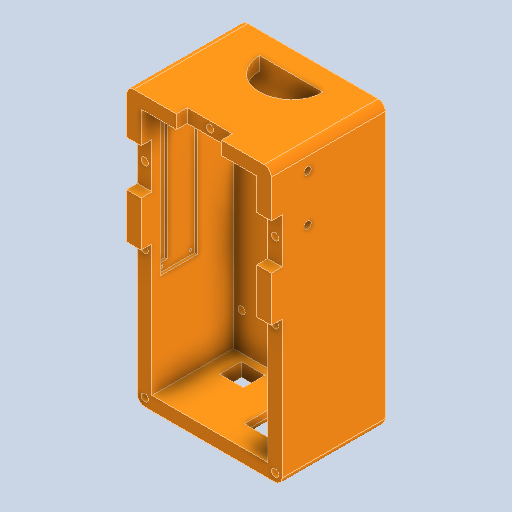
# Autodesk Inventor part: Caja para Electrónica
Saved by Autodesk Inventor 2026 (Build 300175050, 175E)
## iProperties
Created: 2026-02-09
Part Number: Caja para Electrónica
Material: Genérico
Document SubType Name: Modeling
Designer: bello
Density: 1 g/cm^3
Appearance: Naranja
Author: bello
Autodesk Inventor part; units mm, degrees
ref_plane "YZ Plane" through (0, 0, 0) normal (1, 0, 0) x (0, 1, 0)
ref_plane "XZ Plane" through (0, 0, 0) normal (0, 1, 0) x (-1, 0, 0)
ref_plane "XY Plane" through (0, 0, 0) normal (0, 0, 1) x (1, 0, 0)
sketch "Boceto1" plane through (0, 0, 0) normal (0, 0, 1) x (1, 0, 0)
  line L0 (0, 0) -> (80, 0)
  line L1 (80, 0) -> (80, -155)
  line L2 (80, -155) -> (0, -155)
  line L3 (0, -155) -> (0, 0)
  dimension "d0" = 155
  dimension "d1" = 80
  constraints: 8 end point, 2 parallel, 1 horizontal, 1 perpendicular
  measures "d0" distance of L0.end L1.end
  measures "d1" distance of L0.start L0.end
extrude "Extrusión1" add sketch "Boceto1" along normal blind 82
sketch "Boceto2" plane through (0, 0, 82) normal (0, 0, 1) x (1, 0, 0)
  line L0 (8, -7.5) -> (72, -7.5)
  line L1 (72, -7.5) -> (72, -147.5)
  line L2 (72, -147.5) -> (8, -147.5)
  line L3 (8, -147.5) -> (8, -7.5)
  line L4 (80, -155) -> (80, 0) projected
  line L5 (0, 0) -> (0, -155) projected
  line L6 (80, 0) -> (0, 0) projected
  line L7 (0, -155) -> (80, -155) projected
  dimension "d4" = 8
  dimension "d5" = 8
  dimension "d6" = 7.5
  dimension "d7" = 7.5
  dimension "d8" = 64
  dimension "d9" = 140
  constraints: 8 end point, 2 parallel, 1 horizontal, 1 perpendicular
  measures "d4" distance between parallel lines of L4 L1
  measures "d5" distance between parallel lines of L5 L3
  measures "d6" distance between parallel lines of L6 L0
  measures "d7" distance between parallel lines of L7 L2
  measures "d8" distance between parallel lines of L1 L3
  measures "d9" distance between parallel lines of L2 L0
extrude "Extrusión2" cut sketch "Boceto2" against normal blind 70 contours L0 L1 L2 L3
sketch "Boceto3" plane through (0, 0, 12) normal (0, 0, 1) x (1, 0, 0)
  line L0 (72, -147.5) -> (8, -147.5) projected
  line L1 (8, -147.5) -> (8, -7.5) projected
  line L2 (72, -7.5) -> (72, -147.5) projected
  line L3 (10, -142) -> (70, -142)
  circle A0 centre (12.5, -127) radius 2
  circle A1 centre (60.5, -128) radius 2
  circle A2 centre (60.5, -46.5) radius 2
  point P0 (0, 0)
  dimension "d20" = 60
  dimension "d21" = 2
  dimension "d22" = 2
  dimension "d23" = 5.5
  dimension "d24" = 15
  dimension "d25" = 14
  dimension "d26" = 4.5
  dimension "d27" = 11.5
  dimension "d28" = 95.5
  dimension "d29" = 11.5
  dimension "d30" = 4
  constraints: 3 centre point, 2 end point, 2 equal radius, 1 horizontal
  measures "d20" distance of L3.start L3.end
  measures "d21" distance from line of L1 L3.start
  measures "d22" distance from line of L2 L3.end
  measures "d23" distance between parallel lines of L0 L3
  measures "d24" distance from line of L3 A0.centre
  measures "d25" distance from line of L3 A1.centre
  measures "d26" distance from line of L1 A0.centre
  measures "d27" distance from line of L2 A1.centre
  measures "d28" distance from line of L3 A2.centre
  measures "d29" distance from line of L2 A2.centre
  measures "d30" diameter of A2
extrude "Extrusión3" cut sketch "Boceto3" against normal blind 6.7
sketch "Boceto4" plane through (0, 0, 12) normal (0, 0, 1) x (1, 0, 0)
  line L0 (40, 12.201) -> (40, -183.6096)
  circle A0 centre (40, -57.5) radius 3
  circle A1 centre (40, -117.5) radius 3
  line L1 (72, -147.5) -> (8, -147.5) projected
  line L2 (0, -155) -> (80, -155) projected
  point P0 (0, 0)
  point P1 (40, -155)
  point P2 (40, -155)
  dimension "d33" = 60
  dimension "d34" = 6
  dimension "d35" = 30
  dimension "d103" = 0
  constraints: 2 centre point, 2 end point, 2 midpoint, 2 point on line, 1 equal radius
  measures "d33" distance of A1.centre A0.centre
  measures "d34" diameter of A0
  measures "d35" distance from line of L1 A1.centre
  measures "d103" distance from line of point (40, -155) L0
extrude "Extrusión4" cut sketch "Boceto4" against normal through all
sketch "Boceto5" plane through (0, 0, 12) normal (0, 0, 1) x (1, 0, 0)
  circle A0 centre (40, -57.5) radius 3 projected
  line L0 (45.9467, -57.5) -> (42.9734, -62.65)
  line L1 (42.9734, -62.65) -> (37.0266, -62.65)
  line L2 (37.0266, -62.65) -> (34.0533, -57.5)
  line L3 (34.0533, -57.5) -> (37.0266, -52.35)
  line L4 (37.0266, -52.35) -> (42.9734, -52.35)
  line L5 (42.9734, -52.35) -> (45.9467, -57.5)
  circle A1 centre (40, -117.5) radius 3 projected
  line L6 (45.9467, -117.5) -> (42.9734, -122.65)
  line L7 (42.9734, -122.65) -> (37.0266, -122.65)
  line L8 (37.0266, -122.65) -> (34.0533, -117.5)
  line L9 (34.0533, -117.5) -> (37.0266, -112.35)
  line L10 (37.0266, -112.35) -> (42.9734, -112.35)
  line L11 (42.9734, -112.35) -> (45.9467, -117.5)
  point P0 (0, 0)
  dimension "d38" = 10.3
  constraints: 24 end point, 2 coincident, 1 parallel, 26 other
  measures "d38" distance between parallel lines of L1 L4
extrude "Extrusión5" cut sketch "Boceto5" against normal blind 6 contours A0 | L0 L1 L2 L3 L4 L5 | A1 | L6 L7 L8 L9 L10 L11
sketch "Boceto6" plane through (0, -155, 0) normal (0, -1, 0) x (1, 0, 0)
  line L0 (0, 0) -> (80, 0) projected
  line L1 (72, 12) -> (8, 12) projected
  line L2 (16.5, 16) -> (29.5, 16)
  line L3 (16.5, 28) -> (29.5, 28)
  line L4 (10, 12) -> (10, 44.9628)
  line L5 (70, 12) -> (70, 46.4487)
  line L6 (8, 82) -> (8, 12) projected
  line L7 (72, 82) -> (72, 12) projected
  line L8 (16.5, 28) -> (16.5, 16)
  line L9 (29.5, 28) -> (29.5, 16)
  line L10 (47, 45) -> (68.5, 45)
  line L11 (47, 28.5) -> (68.5, 28.5)
  line L12 (47, 28.5) -> (47, 45)
  line L13 (68.5, 28.5) -> (68.5, 45)
  point P0 (23, 16)
  dimension "d41" = 12
  dimension "d42" = 4
  dimension "d43" = 16
  dimension "d44" = 2
  dimension "d45" = 2
  dimension "d46" = 13
  dimension "d47" = 13
  dimension "d48" = 6.5
  dimension "d49" = 6.5
  dimension "d50" = 12
  dimension "d53" = 33
  dimension "d54" = 16.5
  dimension "d55" = 21.5
  dimension "d56" = 1.5
  dimension "d57" = 1.5
  dimension "d58" = 16.5
  constraints: 20 end point, 4 horizontal, 2 point on line, 2 vertical, 1 midpoint, 1 parallel
  measures "d41" distance between parallel lines of L0 L1
  measures "d42" distance between parallel lines of L1 L2
  measures "d43" distance between parallel lines of L1 L3
  measures "d44" distance between parallel lines of L6 L4
  measures "d45" distance between parallel lines of L7 L5
  measures "d46" distance of L3.start L3.end
  measures "d47" distance of L2.start L2.end
  measures "d48" distance from line of L4 L3.start
  measures "d49" distance from line of L4 L2.start
  measures "d50" distance from line of point (23, 16) L3
  measures "d53" distance between parallel lines of L1 L10
  measures "d54" distance between parallel lines of L1 L11
  measures "d55" distance of L10.start L10.end
  measures "d56" distance from line of L5 L10.end
  measures "d57" distance from line of L5 L11.end
  measures "d58" distance between parallel lines of L10 L11
extrude "Extrusión6" cut sketch "Boceto6" against normal up to surface (7.5 mm away)
fillet "Empalme1" radius 4 4 edges at (47, -155, 36.75) (57.75, -155, 45) (68.5, -155, 36.75) (57.75, -155, 28.5)
sketch "Boceto8" plane through (72, -147.5, 82) normal (-1, 0, 0) x (0, 0, 1)
  line L0 (-50, 126.4237) -> (-50, 59.6822)
  line L1 (-70, 0) -> (-70, 140) projected
  circle A0 centre (-39, 136.5) radius 2
  circle A1 centre (-39, 110.5) radius 2
  line L2 (-54.9354, 5.5) -> (-15.6963, 5.5)
  line L3 (0, 0) -> (-70, 0) projected
  line L4 (-50, 108) -> (-15.6963, 108)
  line L5 (-50, 139) -> (-21.6523, 139)
  point P0 (-82, 147.5)
  dimension "d60" = 20
  dimension "d61" = 4
  dimension "d62" = 11
  dimension "d63" = 11
  dimension "d64" = 5.5
  dimension "d65" = 102.5
  dimension "d66" = 2.5
  dimension "d67" = 31
  dimension "d68" = 2.5
  constraints: 8 end point, 3 horizontal, 2 centre point, 2 point on line, 1 equal radius, 1 vertical
  measures "d60" distance between parallel lines of L1 L0
  measures "d61" diameter of A0
  measures "d62" distance from line of A0.centre L0
  measures "d63" distance from line of L0 A1.centre
  measures "d64" distance between parallel lines of L3 L2
  measures "d65" distance between parallel lines of L2 L4
  measures "d66" distance from line of L4 A1.centre
  measures "d67" distance between parallel lines of L4 L5
  measures "d68" distance from line of L5 A0.centre
extrude "Extrusión7" cut sketch "Boceto8" against normal through all
sketch "Boceto9" plane through (8, -147.5, 82) normal (1, 0, 0) x (0, 0, -1)
  line L0 (50, 55) -> (50, 136)
  line L1 (70, 140) -> (70, 0) projected
  line L2 (29.5, 55) -> (29.5, 136)
  line L3 (50, 55) -> (29.5, 55)
  line L4 (29.5, 136) -> (50, 136)
  point P0 (82, 147.5)
  point P1 (0, 140)
  point P2 (39.75, 55)
  dimension "d71" = 20
  dimension "d72" = 20.5
  dimension "d73" = 81
  dimension "d75" = 4
  dimension "d101" = 30.25
  constraints: 8 end point, 2 vertical, 1 horizontal, 1 midpoint, 1 parallel
  measures "d71" distance between parallel lines of L1 L0
  measures "d72" distance between parallel lines of L0 L2
  measures "d73" distance of L2.start L2.end
  measures "d75" vertical distance of point (0, 140) L2.end
  measures "d101" distance from line of L1 point (39.75, 55)
extrude "Extrusión8" cut sketch "Boceto9" against normal blind 1.5
sketch "Boceto10" plane through (6.5, -147.5, 82) normal (1, 0, 0) x (0, 0, -1)
  line L0 (35, 59.5) -> (35, 131.5)
  line L1 (35, 131.5) -> (31, 131.5)
  line L2 (31, 131.5) -> (31, 59.5)
  line L3 (31, 59.5) -> (35, 59.5)
  line L4 (29.5, 55) -> (29.5, 136) projected
  line L5 (29.5, 136) -> (50, 136) projected
  point P0 (82, 147.5)
  point P1 (29.5, 95.5)
  dimension "d79" = 72
  dimension "d80" = 1.5
  dimension "d81" = 4
  dimension "d83" = 36
  constraints: 8 end point, 2 perpendicular, 1 midpoint, 1 parallel, 1 vertical
  measures "d79" distance of L1.end L2.end
  measures "d80" distance between parallel lines of L2 L4
  measures "d81" distance between parallel lines of L0 L2
  measures "d83" distance from line of point (29.5, 95.5) L1
extrude "Extrusión9" cut sketch "Boceto10" against normal blind 1.5
sketch "Boceto11" plane through (6.5, -147.5, 82) normal (1, 0, 0) x (0, 0, -1)
  circle A0 centre (31.75, 57.5) radius 0.8
  circle A1 centre (47.75, 57.5) radius 0.8
  circle A2 centre (31.75, 133.5) radius 0.8
  circle A3 centre (47.75, 133.5) radius 0.8
  line L0 (50, 136) -> (50, 55) projected
  line L1 (50, 55) -> (29.5, 55) projected
  line L2 (29.5, 55) -> (29.5, 136) projected
  line L3 (29.5, 136) -> (50, 136) projected
  point P0 (82, 147.5)
  dimension "d86" = 1.6
  dimension "d88" = 2.25
  dimension "d89" = 2.25
  dimension "d91" = 2.5
  dimension "d92" = 2.25
  dimension "d93" = 2.5
  dimension "d94" = 2.5
  dimension "d95" = 2.5
  dimension "d96" = 2.25
  constraints: 4 centre point, 3 equal radius
  measures "d86" diameter of A0
  measures "d88" distance from line of L0 A1.centre
  measures "d89" distance from line of L0 A3.centre
  measures "d91" distance from line of L1 A0.centre
  measures "d92" distance from line of L2 A0.centre
  measures "d93" distance from line of L1 A1.centre
  measures "d94" distance from line of L3 A3.centre
  measures "d95" distance from line of L3 A2.centre
  measures "d96" distance from line of L2 A2.centre
extrude "Extrusión10" cut sketch "Boceto11" against normal blind 3.5 contours A0 | A1 | A2 | A3
sketch "Boceto12" plane through (0, 0, 82) normal (0, 0, 1) x (1, 0, 0)
  line L0 (0, -75) -> (80, -75)
  line L1 (0, -155) -> (80, -155) projected
  line L2 (0, -75) -> (0, -155)
  line L3 (0, -155) -> (80, -155)
  line L4 (80, -155) -> (80, -75)
  point P0 (0, 0)
  point P1 (40, -155)
  dimension "d99" = 80
  dimension "d100" = 40
  dimension "d104" = 80
  dimension "d105" = 80
  constraints: 8 end point, 2 perpendicular, 1 horizontal, 1 midpoint, 1 vertical
  measures "d99" distance of L0.start L0.end
  measures "d100" horizontal distance of point (40, -155) L0.start
  measures "d104" distance of L3.end L0.end
  measures "d105" distance between parallel lines of L1 L0
extrude "Extrusión11" cut sketch "Boceto12" against normal blind 25
sketch "Boceto13" plane through (8, -7.5, 82) normal (0, -1, 0) x (1, 0, 0)
  line L0 (0, -70) -> (64, -70) projected
  circle A0 centre (32, -70) radius 17.5
  point P0 (-8, -82)
  point P1 (49.5, -70)
  point P2 (14.5, -70)
  dimension "d108" = 35
  constraints: 1 centre point, 1 midpoint
  measures "d108" diameter of A0
extrude "Extrusión12" cut sketch "Boceto13" against normal through all contours A0 L0 picked at (31.4056, -58.945)
sketch "Boceto14" plane through (0, 0, 57) normal (0, 0, 1) x (1, 0, 0)
  circle A0 centre (4, -150.5) radius 2
  circle A1 centre (4, -79.5) radius 2
  circle A2 centre (76, -79.5) radius 2
  circle A3 centre (76, -150.5) radius 2
  line L0 (80, -155) -> (0, -155) projected
  line L1 (0, -155) -> (0, -75) projected
  line L2 (0, -75) -> (8, -75) projected
  line L3 (80, -75) -> (80, -155) projected
  line L4 (72, -75) -> (80, -75) projected
  point P0 (0, 0)
  dimension "d111" = 4
  dimension "d112" = 4.5
  dimension "d113" = 4
  dimension "d114" = 4.5
  dimension "d115" = 4
  dimension "d116" = 4
  dimension "d117" = 4.5
  dimension "d118" = 4
  dimension "d119" = 4.5
  constraints: 4 centre point, 3 equal radius
  measures "d111" diameter of A0
  measures "d112" distance from line of L0 A0.centre
  measures "d113" distance from line of L1 A0.centre
  measures "d114" distance from line of L2 A1.centre
  measures "d115" distance from line of L1 A1.centre
  measures "d116" distance from line of L3 A2.centre
  measures "d117" distance from line of L4 A2.centre
  measures "d118" distance from line of L3 A3.centre
  measures "d119" distance from line of L0 A3.centre
extrude "Extrusión13" cut sketch "Boceto14" against normal blind 6.7
sketch "Boceto15" plane through (0, 0, 82) normal (0, 0, 1) x (1, 0, 0)
  line L0 (0, 0) -> (0, -75) projected
  line L1 (72, -75) -> (80, -75) projected
  line L2 (0, 0) -> (80, 0)
  line L3 (80, 0) -> (80, -75)
  line L4 (80, -75) -> (0, -75)
  line L5 (0, -75) -> (0, 0)
  constraints: 8 end point, 2 parallel, 1 horizontal, 1 perpendicular
extrude "Extrusión14" cut sketch "Boceto15" against normal blind 19
fillet "Empalme2" radius 4 4 edges at (0, -155, 28.5) (80, -155, 28.5) (80, 0, 31.5) (0, 0, 31.5)
sketch "Boceto16" plane through (0, 0, 63) normal (0, 0, 1) x (1, 0, 0)
  line L0 (22.5, 0) -> (57.5, 0) projected
  line L1 (27.5, -7.5) -> (52.5, -7.5)
  line L2 (52.5, -7.5) -> (52.5, 0)
  line L3 (52.5, 0) -> (27.5, 0)
  line L4 (27.5, 0) -> (27.5, -7.5)
  line L5 (8, -147.5) -> (8, -7.5) projected
  line L6 (0, -25) -> (8, -25)
  line L7 (8, -25) -> (8, -50)
  line L8 (8, -50) -> (0, -50)
  line L9 (0, -50) -> (0, -25)
  line L10 (8, -75) -> (0, -75) projected
  line L11 (40, 16.6758) -> (40, -44.6226)
  line L12 (80, -25) -> (72, -25)
  line L13 (72, -25) -> (72, -50)
  line L14 (72, -50) -> (80, -50)
  line L15 (80, -50) -> (80, -25)
  point P0 (40, 0)
  dimension "d129" = 25
  dimension "d130" = 7.5
  dimension "d131" = 12.5
  dimension "d132" = 8
  dimension "d133" = 25
  dimension "d134" = 25
  constraints: 26 end point, 4 parallel, 4 symmetric about line, 2 horizontal, 2 perpendicular, 2 point on line, 1 midpoint, 1 vertical
  measures "d129" distance of L1.start L1.end
  measures "d130" distance of L1.end L2.end
  measures "d131" distance from line of point (40, 0) L4
  measures "d132" distance of L6.start L6.end
  measures "d133" distance of L8.end L6.start
  measures "d134" distance between parallel lines of L10 L8
extrude "Extrusión15" cut sketch "Boceto16" against normal blind 6
sketch "Boceto17" plane through (0, 0, 57) normal (0, 0, 1) x (1, 0, 0)
  circle A0 centre (40, -3.75) radius 2
  circle A1 centre (4, -37.5) radius 2
  line L0 (5, -77.7679) -> (5, -16) projected
  circle A2 centre (76, -37.5) radius 2
  line L1 (0, -50) -> (0, -25) projected
  line L2 (0, -25) -> (8, -25) projected
  line L3 (80, -50) -> (72, -50) projected
  line L4 (80, -25) -> (80, -50) projected
  line L5 (52.5, -7.5) -> (27.5, -7.5) projected
  line L6 (27.5, -7.5) -> (27.5, 0) projected
  point P0 (0, 0)
  dimension "d137" = 4
  dimension "d138" = 4
  dimension "d139" = 12.5
  dimension "d140" = 12.5
  dimension "d141" = 4
  dimension "d142" = 3.75
  dimension "d143" = 12.5
  constraints: 3 centre point, 2 equal radius
  measures "d137" diameter of A0
  measures "d138" distance from line of L1 A1.centre
  measures "d139" distance from line of L2 A1.centre
  measures "d140" distance from line of L3 A2.centre
  measures "d141" distance from line of L4 A2.centre
  measures "d142" distance from line of L5 A0.centre
  measures "d143" distance from line of L6 A0.centre
extrude "Extrusión16" cut sketch "Boceto17" against normal blind 6.7
